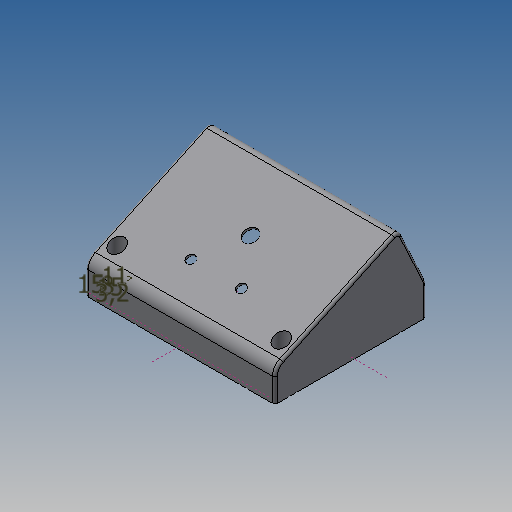
# Autodesk Inventor part: Couvercle_Meca_IIm_Ligne
Saved by Autodesk Inventor 2025.3 (Build 293356000, 356)
## iProperties
Created: 2026-08-27
Part Number: Couvercle_Meca_IIm_Ligne
Project: Nom Projet
Material: .
Description: Nom pièce
Document SubType Name: Modeling
Designer: jules
Authority: brut Ø
Mass: 0.0925188 g
Surface Area: 867.594 cm^2
Volume: 92.5188 cm^3
Density: 0.001 g/cm^3
Appearance: Par défaut
Material number: ---
Author: jules
Autodesk Inventor part; units mm, degrees
ref_plane "Plan YZ" through (0, 0, 0) normal (1, 0, 0) x (0, 1, 0)
ref_plane "Plan XZ" through (0, 0, 0) normal (0, 1, 0) x (-1, 0, 0)
ref_plane "Plan XY" through (0, 0, 0) normal (0, 0, 1) x (1, 0, 0)
sketch "Esquisse1" plane through (0, 0, 0) normal (0, 0, 1) x (1, 0, 0)
  line L0 (75, -60) -> (-75, -60)
  line L1 (-75, -60) -> (-75, 60)
  line L2 (-75, 60) -> (75, 60)
  line L3 (75, 60) -> (75, -60)
  line L4 (75, -60) -> (-75, 60) construction
  line L5 (-75, -60) -> (75, 60) construction
  point P0 (0, 0)
  dimension "d0" = 150
  dimension "d1" = 120
  constraints: 12 end point, 2 midpoint, 2 parallel, 1 horizontal, 1 perpendicular
  measures "d0" distance between parallel lines of L3 L1
  measures "d1" distance between parallel lines of L0 L2
extrude "Extrusion1" add sketch "Esquisse1" along normal blind 25
sketch "Esquisse6" plane through (75, -60, 0) normal (1, 0, 0) x (0, 0, -1)
  line L0 (-25, 0) -> (-25, 120) projected
  line L1 (-25, 0) -> (-70.9627, 98.5673)
  line L2 (-70.9627, 98.5673) -> (-25, 120)
  point P0 (0, 60)
  dimension "d4" = 25
  constraints: 4 end point, 1 perpendicular
  measures "d4" angle of L0 L1
extrude "Extrusion2" add sketch "Esquisse6" against normal up to surface (150 mm away)
shell "Coque1" thickness 2 removed faces 1 at (-25, -20, 0)
fillet "Congé1" radius 10 4 edges at (0, 58, 24.5566) (0, -58, 23.7259) (0, -60, 25) (0, 60, 25)
sketch "Esquisse7" plane through (-75, 60, 0) normal (0, 1, 0) x (1, 0, 0)
  line L0 (150, 0) -> (0, 0) projected
  line L1 (-30, 0) -> (180, 0) construction
  line L2 (75, 14.1925) -> (75, -85.1552) construction
  line L3 (130, 0) -> (130, -20)
  line L4 (130, -20) -> (75, -20)
  line L5 (20, 0) -> (20, -20)
  line L6 (20, -20) -> (75, -20)
  point P0 (75, 0)
  dimension "d9" = 20
  dimension "d10" = 110
  constraints: 8 end point, 2 point on line, 2 symmetric about line, 1 perpendicular, 1 vertical
  measures "d9" distance between parallel lines of L0 L4
  measures "d10" distance between parallel lines of L5 L3
extrude "Extrusion3" cut sketch "Esquisse7" against normal up to surface (2 mm away)
fillet "Congé2" radius 5 4 edges at (55, 59, 20) (55, 59, 0) (-55, 59, 20) (-55, 59, 0)
fillet "Congé3" radius 5 2 edges at (0, 38.5673, 70.9627) (0, 37.5999, 68.3048)
fillet "Congé4" radius 2 14 edges at (-75, -58.4339, 24.0023) (-75, -10.0952, 48.271) (-75, 37.8589, 69.0165) (-75, 49.8717, 46.7202) (-75, 59.763, 24.9474) (-75, 60, 11.3915) (-75, -60, 9.3146) (75, -58.4339, 24.0023) (75, -10.0952, 48.271) (75, 37.8589, 69.0165) (75, 49.8717, 46.7202) (75, 59.763, 24.9474) (75, 60, 11.3915) (75, -60, 9.3146)
sketch "Esquisse8" plane through (-73, 34.0357, 68.8496) normal (0, -0.4226183, 0.9063078) x (1, 0, 0)
  line L0 (0, -97.3862) -> (146, -97.3862) construction
  line L1 (146, -97.3862) -> (146, -17.3862) construction
  line L2 (146, -17.3862) -> (0, -17.3862) construction
  line L3 (0, -17.3862) -> (0, -97.3862) construction
  line L4 (0, -97.3862) -> (146, -17.3862) construction
  line L5 (146, -97.3862) -> (0, -17.3862) construction
  line L6 (146, -97.3862) -> (0, -97.3862) construction
  line L7 (146, 0) -> (146, -97.3862) construction
  line L8 (45.625, -72.3862) -> (100.375, -72.3862) construction
  circle A0 centre (53, -72.3862) radius 3.5 construction
  line L9 (73, -141.9328) -> (73, 51.34) construction
  circle A1 centre (93, -72.3862) radius 3.5 construction
  line L10 (27.375, -82.3862) -> (118.625, -82.3862) construction
  circle A2 centre (73, -42.3862) radius 5.5 construction
  circle A3 centre (10, -17.3862) radius 3 construction
  circle A4 centre (30, -17.3862) radius 1.5 construction
  circle A5 centre (53, -82.3862) radius 1.5 construction
  circle A6 centre (93, -82.3862) radius 1.5 construction
  point P0 (73, -57.3862)
  point P1 (73, -57.3862)
  dimension "d16" = 146
  dimension "d17" = 80
  dimension "d27" = 7
  dimension "d28" = 40
  dimension "d29" = 10
  dimension "d37" = 15
  dimension "d38" = 11
  dimension "d39" = 15
  dimension "d73" = 6
  dimension "d74" = 10
  dimension "d75" = 3
  dimension "d76" = 20
  dimension "d77" = 3
  dimension "d78" = 40
  constraints: 16 end point, 9 point on line, 7 centre point, 4 parallel, 2 collinear, 2 midpoint, 2 symmetric about line, 1 horizontal, 1 perpendicular, 2 other
  measures "d16" distance of L2.end L1.end
  measures "d17" distance between parallel lines of L0 L2
  measures "d27" diameter of A0
  measures "d28" distance of A1.centre A0.centre
  measures "d29" distance between parallel lines of L10 L8
  measures "d37" distance from line of L8 point (73, -57.386)
  measures "d38" diameter of A2
  measures "d39" distance of point (73, -57.386) A2.centre
  measures "d73" diameter of A3
  measures "d74" distance from line of L3 A3.centre
  measures "d75" diameter of A4
  measures "d76" distance of A3.centre A4.centre
  measures "d77" diameter of A5
  measures "d78" distance of A6.centre A5.centre
hole "Perçage1" at (0, -4.3793, 50.9364) direction (0, 0.4226183, -0.9063078) diameter 11 end through all start extended yes clearance for "Vis à tête plate fraisée ISO 2009/7046" size "M10" standard "ISO"
hole "Perçage2" at (-20, -31.5685, 38.2578) at (20, -31.5685, 38.2578) direction (0, 0.4226183, -0.9063078) diameter 7 end through all start extended yes
sketch "Esquisse9" plane through (0, 0, 0) normal (0, 0, -1) x (-1, 0, 0)
  line L0 (73, -58) -> (-73, -58) construction
  line L1 (73, 58) -> (73, -58) construction
  line L2 (60, 58) -> (73, 58) construction
  line L3 (60, 58) -> (60, 60) construction
  line L4 (60, 60) -> (73, 60) construction
  line L5 (-73, 60) -> (-60, 60) construction
  line L6 (-73, 58) -> (-60, 58) construction
  line L7 (-60, 60) -> (-60, 58) construction
  line L8 (-73, -58) -> (-73, 58) construction
  line L9 (-60, 58) -> (-73, 58)
  line L10 (-73, 58) -> (-73, -58)
  line L11 (-73, -58) -> (73, -58)
  line L12 (73, -58) -> (73, 58)
  line L13 (60, 58) -> (73, 58)
  line L14 (60, 58) -> (60, 59.1)
  line L15 (60, 59.1) -> (74.1, 59.1)
  line L16 (74.1, 59.1) -> (74.1, -59.1)
  line L17 (74.1, -59.1) -> (-74.1, -59.1)
  line L18 (-74.1, -59.1) -> (-74.1, 59)
  line L19 (-74.1, 59) -> (-60, 59)
  line L20 (-60, 58) -> (-60, 59)
  point P0 (0, 0)
  dimension "d40" = 1.1
  dimension "d41" = 1.1
  dimension "d42" = 1.1
  dimension "d43" = 1.1
  constraints: 24 end point, 6 perpendicular, 3 collinear, 2 parallel, 2 point on line, 1 midpoint
  measures "d40" distance of L2.start L14.end
  measures "d41" distance between parallel lines of L18 L8
  measures "d42" distance between parallel lines of L12 L16
  measures "d43" distance between parallel lines of L0 L17
extrude "Extrusion4" cut sketch "Esquisse9" against normal blind 1.2
fillet "Congé5" radius 2 4 edges at (-74.1, -59.1, 0.6) (-74.1, 59.1, 0.6) (74.1, -59.1, 0.6) (74.1, 59, 0.6)
sketch "Esquisse10" plane through (50, 60, 20) normal (0, 0, -1) x (-1, 0, 0)
  line L0 (50, -144) -> (50, 24) construction
  line L1 (100, -2) -> (0, -2) construction
  line L2 (19.75, -2) -> (19.75, -0.9)
  line L3 (123, -0.9369) -> (-23, -0.9369) construction
  line L4 (19.75, -0.9) -> (80.25, -0.9)
  line L5 (80.25, -0.9) -> (80.25, -2)
  line L6 (19.75, -2) -> (80.25, -2)
  point P0 (50, -60)
  point P1 (50, -0.9)
  dimension "d47" = 1.1
  dimension "d48" = 60.5
  constraints: 8 end point, 3 point on line, 2 perpendicular, 1 collinear, 1 midpoint, 1 parallel
  measures "d47" distance between parallel lines of L1 L4
  measures "d48" distance between parallel lines of L2 L5
extrude "Extrusion5" cut sketch "Esquisse10" against normal blind 1.2
ref_plane "Plan de construction1" through (0, 0, 3) normal (0, 0, -1) x (-1, 0, 0)
sketch "Esquisse12" plane through (0, 0, 3) normal (0, 0, -1) x (-1, 0, 0)
  line L0 (73, -58) -> (73, 58) construction
  line L1 (-73, -58) -> (73, -58) construction
  line L2 (-73, 58) -> (-73, -58) construction
  line L3 (73, -52.5) -> (65, -52.5)
  line L4 (73, -52.5) -> (73, -37.5)
  line L5 (73, -37.5) -> (65, -37.5)
  arc A0 (65, -37.5) -> (65, -52.5) centre (65, -45) ccw
  circle A1 centre (65, -45) radius 1.6 construction
  circle A2 centre (65, -45) radius 5.5 construction
  line L6 (73, -60) -> (-73, -60) construction
  line L7 (105, 0) -> (-105, 0) construction
  line L8 (0, -84) -> (0, 84) construction
  line L9 (73, 52.5) -> (65, 52.5)
  line L10 (73, 52.5) -> (73, 37.5)
  line L11 (73, 37.5) -> (65, 37.5)
  arc A3 (65, 52.5) -> (65, 37.5) centre (65, 45) ccw
  circle A4 centre (65, 45) radius 1.6 construction
  circle A5 centre (65, 45) radius 5.5 construction
  line L12 (-73, -52.5) -> (-65, -52.5)
  line L13 (-73, -52.5) -> (-73, -37.5)
  line L14 (-73, -37.5) -> (-65, -37.5)
  arc A6 (-65, -52.5) -> (-65, -37.5) centre (-65, -45) ccw
  circle A7 centre (-65, -45) radius 1.6 construction
  circle A8 centre (-65, -45) radius 5.5 construction
  line L15 (-73, 52.5) -> (-65, 52.5)
  arc A9 (-65, 37.5) -> (-65, 52.5) centre (-65, 45) ccw
  circle A10 centre (-65, 45) radius 5.5 construction
  circle A11 centre (-65, 45) radius 1.6 construction
  line L16 (-73, 37.5) -> (-65, 37.5)
  line L17 (-73, 52.5) -> (-73, 37.5)
  point P0 (0, 0)
  dimension "d52" = 3.2
  dimension "d53" = 11
  dimension "d54" = 15
  dimension "d55" = 8
  dimension "d56" = 15
  constraints: 24 end point, 21 symmetric about line, 12 centre point, 8 coincident, 8 point on circle, 2 horizontal, 2 point on line, 2 tangent, 9 other
  measures "d52" diameter of A1
  measures "d53" diameter of A2
  measures "d54" distance between parallel lines of L3 L5
  measures "d55" distance from line of L0 A0.centre
  measures "d56" distance from line of L6 A0.centre
extrude "Extrusion6" add sketch "Esquisse12" against normal up to surface contours L3 A0 L5 L4 surface through (75, -59.1548, 23.1874) normal (0, -0.4226183, 0.9063078)
ref_plane "Plan de construction2" through (0, 0, 5) normal (0, 0, -1) x (-1, 0, 0)
extrude "Extrusion7" add sketch "Esquisse12" against normal up to surface contours L10 L11 A3 L9 surface through (75, 36.7546, 70.1174) normal (0, 0.9063078, 0.4226183)
extrude "Extrusion8" add sketch "Esquisse12" against normal up to surface contours L15 A9 L16 L17 surface through (75, 36.7546, 70.1174) normal (0, 0.9063078, 0.4226183)
extrude "Extrusion9" add sketch "Esquisse12" against normal up to surface contours L13 L14 A6 L12 surface through (75, -59.1548, 23.1874) normal (0, -0.4226183, 0.9063078)
sketch "Esquisse13" plane through (0, 0, 5) normal (0, 0, -1) x (-1, 0, 0)
  point P0 (0, 0)
  point P1 (65, -45)
  point P2 (65, 45)
  point P3 (-65, 45)
  point P4 (-65, -45)
hole "Perçage3" at (-65, -45, 5) at (65, -45, 5) at (65, 45, 5) at (-65, 45, 5) direction (0, 0, -1) diameter 3.4 depth 8 start extended yes counterbore diameter 11.5 counterbore depth 0.1 clearance for "Vis d'assemblage à tête hexagonale ISO 24017" size "M3" standard "ISO"
equation "\"d78\" = d28"
